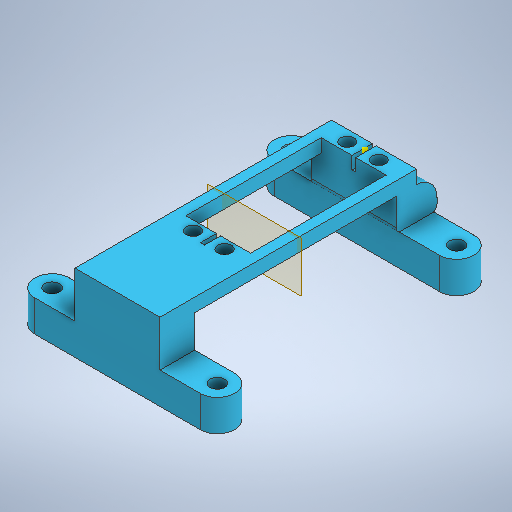
# Autodesk Inventor part: SERVO_MOUNT_TOBASE
Saved by Autodesk Inventor 2025.1 (Build 291241000, 241)
## iProperties
Created: 2024-10-23
Part Number: SERVO_MOUNT_TOBASE
Material: Generic
Document SubType Name: Modeling
Designer: m_kni
Density: 1 g/cm^3
Appearance: Default
Author: m_kni
Autodesk Inventor part; units mm, degrees
ref_plane "YZ Plane" through (0, 0, 0) normal (1, 0, 0) x (0, 1, 0)
ref_plane "XZ Plane" through (0, 0, 0) normal (0, 1, 0) x (-1, 0, 0)
ref_plane "XY Plane" through (0, 0, 0) normal (0, 0, 1) x (1, 0, 0)
sketch "Sketch1" plane through (0, 0, 0) normal (0, 1, 0) x (-1, 0, 0)
  circle A0 centre (-26.1551, -3.0475) radius 2.3
  arc A1 (-34.9051, -0.0475) -> (-17.4051, -0.0475) centre (-26.1551, -0.0475) ccw
  arc A2 (17.5949, -0.0475) -> (35.0949, -0.0475) centre (26.3449, -0.0475) ccw
  circle A3 centre (26.3449, -3.0475) radius 2.3
  circle A4 centre (-26.1551, -3.0475) radius 2.3
  circle A5 centre (26.3449, -3.0475) radius 2.3
  circle A6 centre (26.3449, -0.0475) radius 8.75
  circle A7 centre (-26.1551, -0.0475) radius 8.75
  line L0 (-34.9051, -0.0475) -> (-17.4051, -0.0475)
  line L1 (17.5949, -0.0475) -> (35.0949, -0.0475)
  circle A8 centre (-26.1551, -3.0475) radius 5.5
  circle A9 centre (26.3449, -3.0475) radius 5.5
  line L2 (-26.1551, -8.5475) -> (26.3449, -8.5475)
  line L3 (-26.1551, 2.4525) -> (26.3449, 2.4525)
  point P0 (0, 0)
  dimension "d0" = 11
  dimension "d1" = 11
  dimension "d41" = 4.6
  dimension "d42" = 4.6
  constraints: 9 centre point, 8 end point, 8 point on circle, 6 coincident, 3 concentric, 2 tangent, 1 collinear, 1 horizontal, 1 horizontal alignment, 3 other
  measures "d0" diameter of A8
  measures "d1" diameter of A9
  measures "d41" diameter of A5
  measures "d42" diameter of A4
extrude "Extrusion1" add sketch "Sketch1" along normal blind 10 contours L2 A8 L0 A1 | A1 A7 L3 A6 A2 L2 | A7 L0 A8 L3 | A8 L0 | L0 A8 | A2 L1 A9 L2 | L3 A9 L1 A6 | A9 L1 | A9 L1 picked at (-18.6939, -1.0014) picked at (-20.5799, 1.133) picked at (18.8536, -1.0809) picked at (20.7697, 1.133)
sketch "Sketch2" plane through (0, 10, 0) normal (0, 1, 0) x (1, 0, 0)
  line L0 (26.1551, 8.5475) -> (-26.3449, 8.5475) projected
  line L1 (-26.3449, -2.4525) -> (26.1551, -2.4525) projected
  arc A0 (-26.3449, 8.5475) -> (-26.3449, -2.4525) centre (-26.3449, 3.0475) ccw projected
  arc A1 (26.1551, -2.4525) -> (26.1551, 8.5475) centre (26.1551, 3.0475) ccw projected
  line L2 (-31.8449, 3.0475) -> (31.6551, 3.0475)
  line L3 (13.4051, -3.4525) -> (-13.5949, -3.4525)
  line L4 (-13.5949, -3.4525) -> (-13.5949, 9.5475)
  line L5 (-13.5949, 9.5475) -> (13.4051, 9.5475)
  line L6 (13.4051, 9.5475) -> (13.4051, -3.4525)
  line L7 (13.4051, -3.4525) -> (-13.5949, 9.5475) construction
  line L8 (-13.5949, -3.4525) -> (13.4051, 9.5475) construction
  point P0 (0, 0)
  point P1 (-0.0949, 3.0475)
  dimension "d4" = 27
  dimension "d5" = 13
  constraints: 14 end point, 3 midpoint, 2 parallel, 2 point on circle, 1 horizontal, 1 perpendicular
  measures "d4" distance of L4.end L5.end
  measures "d5" distance of L3.end L4.end
extrude "Extrusion2" add sketch "Sketch2" along normal blind 14.56 contours L6 L2 L4 L0 | L0 L4 L5 L6 | L6 L1 L4 L2 | L6 L3 L4 L1
fillet "Fillet1" radius 2 2 edges at (-0.0949, 10, 3.4525) (-0.0949, 10, -9.5475)
sketch "Sketch3" plane through (0, 24.56, 0) normal (0, 1, 0) x (1, 0, 0)
  arc A0 (-6.4637, 1.2055) -> (-3.8927, 1.3299) centre (-5.0949, -0.4525) ccw
  arc A1 (3.5363, 1.2055) -> (6.1073, 1.3299) centre (4.9051, -0.4525) ccw
  circle A2 centre (4.9051, -0.4525) radius 2.15
  circle A3 centre (-5.0949, -0.4525) radius 2.15
  line L0 (-13.5949, 9.5475) -> (-13.5949, -3.4525) projected
  line L1 (13.4051, 9.5475) -> (-13.5949, 9.5475) projected
  line L2 (-13.5949, -3.4525) -> (13.4051, -3.4525) projected
  line L3 (13.4051, -3.4525) -> (13.4051, 9.5475) projected
  point P0 (0, 0)
  point P1 (6.1073, 1.3299)
  point P2 (3.5363, 1.2055)
  point P3 (-3.8927, 1.3299)
  point P4 (-6.4637, 1.2055)
  dimension "d12" = 8.5
  dimension "d13" = 8.5
  dimension "d43" = 2.15
  dimension "d44" = 2.15
  constraints: 4 centre point, 4 point on circle, 2 coincident, 2 concentric
  measures "d12" distance from line of L0 A0.centre
  measures "d13" distance from line of L3 A1.centre
  measures "d43" radius of A0
  measures "d44" radius of A1
extrude "Extrusion3" cut sketch "Sketch3" against normal blind 10 contours A3 A0 | A2 A1
sketch "Sketch4" plane through (0, 24.56, 0) normal (0, 1, 0) x (1, 0, 0)
  line L0 (13.4051, 9.5475) -> (-13.5949, 9.5475) projected
  line L1 (-13.5949, -2.4525) -> (-13.5949, 8.5475) projected
  line L2 (13.4051, 9.5475) -> (-13.5949, 9.5475)
  line L3 (-13.5949, 9.5475) -> (-13.5949, 3.0475)
  line L4 (-13.5949, 3.0475) -> (13.4051, 3.0475)
  line L5 (13.4051, 3.0475) -> (13.4051, 9.5475)
  point P0 (0, 0)
  constraints: 8 end point, 2 parallel, 1 horizontal, 1 midpoint, 1 perpendicular
extrude "Extrusion4" cut sketch "Sketch4" against normal blind 4.2875
fillet "Fillet2" radius 6.7625 1 edges at (-0.0949, 20.2725, -9.5475)
sketch "Sketch5" plane through (0, 24.56, 0) normal (0, 1, 0) x (1, 0, 0)
  line L0 (-13.5949, -3.4525) -> (13.4051, -3.4525) projected
  line L1 (-10.3949, -3.4525) -> (-10.3949, -67.4525)
  line L2 (10.2051, -3.4525) -> (10.2051, -67.4525)
  line L3 (-13.5949, 3.0475) -> (-13.5949, -3.4525) projected
  circle A0 centre (-5.0949, -49.4525) radius 2.15
  line L4 (13.4051, -3.4525) -> (13.4051, 3.0475) projected
  circle A1 centre (4.9051, -49.4525) radius 2.15
  circle A2 centre (4.9051, -49.4525) radius 3
  circle A3 centre (-5.0949, -49.4525) radius 3
  line L5 (-10.3949, -67.4525) -> (10.2051, -67.4525)
  line L6 (-10.3949, -67.4525) -> (-13.5949, -67.4525)
  line L7 (-13.5949, -67.4525) -> (-13.5949, -3.4525)
  line L8 (10.2051, -67.4525) -> (13.4051, -67.4525)
  line L9 (13.4051, -67.4525) -> (13.4051, -3.4525)
  line L10 (-5.0949, -46.4525) -> (4.9051, -46.4525)
  line L11 (10.2051, -46.4525) -> (-10.3949, -46.4525)
  line L12 (-0.65, -46.4525) -> (-0.65, -51.4525)
  line L13 (-0.65, -51.4525) -> (0.65, -51.4525)
  line L14 (0.65, -51.4525) -> (0.65, -46.4525)
  line L15 (0, -46.4525) -> (-0.65, -51.4525) construction
  line L16 (0, -46.4525) -> (0.65, -51.4525) construction
  point P0 (0, 0)
  point P1 (13.4051, -0.2025)
  point P2 (4.9051, -46.4525)
  dimension "d28" = 6
  dimension "d29" = 6
  dimension "d19" = 3.2
  dimension "d20" = 64
  dimension "d21" = 3.2
  dimension "d22" = 64
  dimension "d23" = 46
  dimension "d24" = 8.5
  dimension "d25" = 4.3
  dimension "d26" = 8.5
  dimension "d27" = 4.3
  dimension "d30" = 1.3
  constraints: 28 end point, 9 point on line, 4 coincident, 4 horizontal, 2 centre point, 2 collinear, 2 vertical, 2 vertical alignment, 1 midpoint, 1 parallel, 4 other
  measures "d19" distance of L1.start L0.start
  measures "d20" distance of L1.start L1.end
  measures "d21" distance of L2.start L0.end
  measures "d22" distance of L2.start L2.end
  measures "d23" distance from line of L0 point (-5.095, -49.453)
  measures "d24" distance from line of L3 point (-5.095, -49.453)
  measures "d25" diameter of A0
  measures "d26" horizontal distance of point (13.405, -0.203) point (4.905, -49.453)
  measures "d27" diameter of A1
  measures "d30" distance of L13.end L12.end
extrude "Extrusion5" add sketch "Sketch5" against normal blind 4.2875 contours L0 L1 L6 L7 | L0 L9 L8 L2 | A2 | A3 | L11 L10 L12 L13 L14 L2 L5 L1
sketch "Sketch6" plane through (0, 24.56, 0) normal (0, 1, 0) x (1, 0, 0)
  line L0 (13.4051, -67.4525) -> (-13.5949, -67.4525) projected
  line L1 (-13.5949, -67.4525) -> (13.4051, -67.4525)
  line L2 (13.4051, -67.4525) -> (13.4051, -78.4525)
  line L3 (13.4051, -78.4525) -> (-13.5949, -78.4525)
  line L4 (-13.5949, -78.4525) -> (-13.5949, -67.4525)
  circle A0 centre (26.1551, 3.0475) radius 2.3 projected
  circle A1 centre (-26.3449, 3.0475) radius 2.3 projected
  point P0 (0, 0)
  dimension "d34" = 11
  constraints: 8 end point, 2 parallel, 1 horizontal, 1 perpendicular
  measures "d34" distance of L1.end L2.end
extrude "Extrusion6" add sketch "Sketch6" against normal up to surface (14.56 mm away) contours L2 L3 L4 L0
ref_plane "Work Plane1" through (-13.5949, 24.56, 34.9525) normal (0, 0, 1) x (1, 0, 0)
sketch "Sketch7" plane through (0, 24.56, 0) normal (0, 1, 0) x (1, 0, 0)
  point P0 (0, 0)
mirror "Mirror1" about plane through (-13.5949, 24.56, 34.9525) normal (0, 0, 1) of "Extrusion1"
sketch "Sketch8" plane through (0, 24.56, 0) normal (0, 1, 0) x (1, 0, 0)
  line L0 (0.6, -3.9565) -> (-0.6, -3.9565)
  line L1 (-0.6, -3.9565) -> (-0.6, 3.9565)
  line L2 (-0.6, 3.9565) -> (0.6, 3.9565)
  line L3 (0.6, 3.9565) -> (0.6, -3.9565)
  line L4 (0.6, -3.9565) -> (-0.6, 3.9565) construction
  line L5 (-0.6, -3.9565) -> (0.6, 3.9565) construction
  point P0 (0, 0)
  dimension "d38" = 1.2
  constraints: 12 end point, 2 midpoint, 2 parallel, 1 horizontal, 1 perpendicular
  measures "d38" distance of L1.end L2.end
extrude "Extrusion7" cut sketch "Sketch8" against normal blind 4
body "Solid1"
